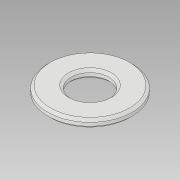
# Autodesk Inventor part: FALSA ARANDELA
Saved by Autodesk Inventor 2019 (Build 230136000, 136)
## iProperties
Created: 2020-04-10
Part Number: FALSA ARANDELA
Material: Plástico ABS
Document SubType Name: Modeling
Designer: Luis Pujol
Density: 1.06 g/cm^3
Appearance: Suave - Blanco
Author: Luis Pujol
Autodesk Inventor part; units mm, degrees
ref_plane "YZ Plane" through (0, 0, 0) normal (1, 0, 0) x (0, 1, 0)
ref_plane "XZ Plane" through (0, 0, 0) normal (0, 1, 0) x (-1, 0, 0)
ref_plane "XY Plane" through (0, 0, 0) normal (0, 0, 1) x (1, 0, 0)
sketch "Boceto1" plane through (0, 0, 0) normal (0, 1, 0) x (-1, 0, 0)
  circle A0 centre (0, 0) radius 5
  circle A1 centre (0, 0) radius 2.25
  dimension "d0" = 10
  dimension "d1" = 4.5
  constraints: 2 centre point, 2 coincident
  measures "d0" diameter of A0
  measures "d1" diameter of A1
extrude "Extrusión1" add sketch "Boceto1" along normal blind 1
chamfer "Chaflán1" distance 0.3 angle 45 4 edges at (2.25, 1, 0) (2.25, 0, 0) (5, 1, 0) (5, 0, 0)
